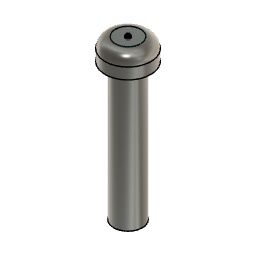
Trammel Toy Assembly (Autodesk Fusion 360 archive; units mm, degrees)
design "Screw"
Autodesk Fusion 360 part; units mm, degrees
sketch "Sketch1" plane through (0, 0, 0) normal (0, 0, 1) x (1, 0, 0)
  circle A0 centre (6.3408, 6.3573) radius 2.1209
  dimension "d1" = 4.2418
  measures "d1" diameter of A0
extrude "Extrude1" add sketch "Sketch1" along normal blind 20.32
sketch "Sketch6" plane through (0, 0, 20.32) normal (0, 0, 1) x (-1, 0, 0)
  circle A0 centre (-6.3408, -6.3573) radius 2.1209
  circle A1 centre (-6.3408, -6.3573) radius 3.3909
  point P0 (-6.3408, -6.3573)
  dimension "d7" = 6.7818
  constraint concentric A0 A1
  measures "d7" diameter of A1
extrude "Extrude2" add sketch "Sketch6" along normal blind 3.175 contours A0 | A1
fillet "Fillet1" radius 1.524 1 edges at (9.5022, 7.5835, 23.495)
sketch "Sketch7" plane through (0, 0, 23.495) normal (0, 0, 1) x (-1, 0, 0)
  circle A0 centre (-6.3408, -6.3573) radius 1.8669
  point P0 (-6.3408, -6.3573)
  constraint coincident P0 A0.centre

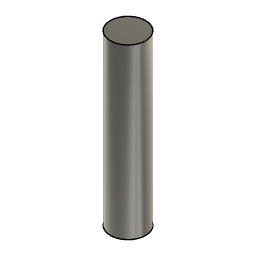
design "PIN"
Autodesk Fusion 360 part; units mm, degrees
sketch "Sketch1" plane through (0, 0, 0) normal (0, 0, 1) x (1, 0, 0)
  circle A0 centre (6.3408, 6.3573) radius 2.1209
  dimension "d1" = 4.2418
  measures "d1" diameter of A0
extrude "Extrude1" add sketch "Sketch1" along normal blind 20.32

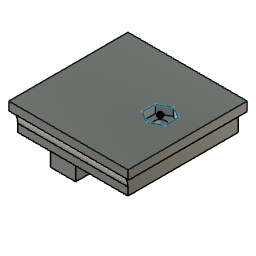
design "Trammel T1 v0"
Autodesk Fusion 360 part; units mm, degrees
sketch "Sketch1" plane through (0, 0, 0) normal (0, 0, 1) x (1, 0, 0)
  line L0 (0, 0) -> (53.975, 0)
  line L1 (53.975, 0) -> (53.975, 53.975)
  line L2 (53.975, 53.975) -> (0, 53.975)
  line L3 (0, 53.975) -> (0, 0)
  dimension "d1" = 53.975
  dimension "d2" = 53.975
  constraint horizontal L0
  constraint vertical L1
  constraint horizontal L2
  constraint vertical L3
  constraint coincident L0.start L3.end
  measures "d1" distance of L0.start L2.end
  measures "d2" distance of L0.start L0.end
extrude "Extrude1" add sketch "Sketch1" along normal blind 12.7
sketch "Sketch2" plane through (53.975, 0, 0) normal (1, 0, 0) x (0, 1, 0)
  line L0 (0, 0) -> (53.975, 0)
  line L1 (53.975, 0) -> (53.975, 12.7)
  line L2 (53.975, 12.7) -> (0, 12.7)
  line L3 (0, 12.7) -> (0, 0)
  line L4 (5.9309, 12.7) -> (0, 12.7)
  line L5 (0, 0) -> (0, 12.7)
  line L6 (0, 0) -> (9.5123, 0)
  line L7 (9.5123, 0) -> (9.5123, 3.175)
  line L8 (5.9309, 9.2761) -> (5.9309, 12.7)
  arc A0 (9.5123, 3.175) -> (5.9309, 9.2761) centre (2.5249, 3.175) ccw
  point P0 (5.9309, 12.7)
  point P1 (9.5123, 0)
  point P2 (9.5123, 3.175)
  point P3 (5.9309, 9.2761)
  dimension "d5" = 5.9309
  dimension "d6" = 9.5123
  dimension "d7" = 3.175
  dimension "d8" = 3.4239
  constraint coincident L2 P0
  constraint coincident L0.start L3.end
  constraint coincident L0 P1
  constraint coincident P0 L4.start
  constraint coincident L2.end L3.start
  constraint coincident P1 L6.end
  constraint coincident P2 L7.end
  constraint perpendicular L6 L7
  constraint coincident P3 L8.start
  constraint perpendicular L2 L8
  constraint tangent L7 A0
  measures "d5" distance of L2.end P0
  measures "d6" distance of L0.start P1
  measures "d7" distance of P1 P2
  measures "d8" distance of P0 P3
extrude "Extrude2" cut sketch "Sketch2" against normal blind 53.975 contours L0 L2 L3 L4 L5 L6 L7 L8 A0
sketch "Sketch3" plane through (0, 53.975, 0) normal (0, 1, 0) x (-1, 0, 0)
  line L0 (-53.975, 0) -> (0, 0)
  line L1 (0, 0) -> (0, 12.7)
  line L2 (0, 12.7) -> (-53.975, 12.7)
  line L3 (-53.975, 12.7) -> (-53.975, 0)
  line L4 (-48.0441, 12.7) -> (-53.975, 12.7)
  line L5 (-53.975, 0) -> (-44.4627, 0)
  line L6 (-44.4627, 9.017) -> (-44.4627, 0)
  line L7 (-44.4627, 9.017) -> (-48.0441, 9.017)
  line L8 (-48.0441, 9.017) -> (-48.0441, 12.7)
  point P0 (-48.0441, 12.7)
  point P1 (-44.4627, 0)
  point P2 (-44.4627, 9.017)
  point P3 (-48.0441, 12.7)
  point P4 (-44.4627, 9.017)
  point P5 (-48.0441, 9.017)
  dimension "d11" = 5.9309
  dimension "d12" = 9.5123
  dimension "d13" = 9.017
  constraint coincident L2 P3
  constraint coincident L0 P1
  constraint coincident P3 P0
  constraint coincident P4 P2
  constraint coincident L2.end L3.start
  constraint coincident L0.start L3.end
  constraint coincident P1 L5.end
  constraint perpendicular L5 L6
  constraint coincident P5 L7.end
  constraint perpendicular L6 L7
  constraint perpendicular L4 L8
  measures "d11" distance of L2.end P3
  measures "d12" distance of L0.start L5.end
  measures "d13" distance of P1 P4
extrude "Extrude3" cut sketch "Sketch3" against normal blind 53.975 contours L0 L2 L3 L4 L5 L6 L7 L8
sketch "Sketch4" plane through (0, 0, 0) normal (0, 0, -1) x (1, 0, 0)
  line L0 (44.4627, -53.975) -> (44.4627, -9.5123)
  line L1 (44.4627, -9.5123) -> (0, -9.5123)
  line L2 (0, -9.5123) -> (0, -53.975)
  line L3 (0, -53.975) -> (44.4627, -53.975)
  line L4 (12.7, -53.975) -> (22.86, -53.975)
  line L5 (22.86, -53.975) -> (22.86, -10.033)
  line L6 (22.86, -10.033) -> (12.7, -10.033)
  line L7 (12.7, -10.033) -> (12.7, -53.975)
  dimension "d16" = 43.942
  dimension "d17" = 10.16
  dimension "d18" = 12.7
  constraint horizontal L4
  constraint vertical L5
  constraint horizontal L6
  constraint vertical L7
  constraint coincident L3 L4.start
  measures "d16" distance of L4.start L6.end
  measures "d17" distance of L4.start L4.end
  measures "d18" distance of L2.end L4.start
sketch "Sketch5" plane through (0, 0, 12.7) normal (0, 0, 1) x (-1, 0, 0)
  line L0 (-48.0441, -5.9309) -> (-48.0441, -53.975)
  line L1 (-48.0441, -53.975) -> (0, -53.975)
  line L2 (0, -53.975) -> (0, -5.9309)
  line L3 (0, -5.9309) -> (-48.0441, -5.9309)
  line L4 (-39.9669, -34.292) -> (-35.3441, -36.9609)
  line L5 (-35.3441, -36.9609) -> (-30.7213, -34.292)
  line L6 (-30.7213, -34.292) -> (-30.7213, -28.954)
  line L7 (-30.7213, -28.954) -> (-35.3441, -26.2851)
  line L8 (-35.3441, -26.2851) -> (-39.9669, -28.954)
  line L9 (-39.9669, -28.954) -> (-39.9669, -34.292)
  point P0 (-35.3441, -31.623)
  point P1 (-35.3441, -31.623)
  dimension "d30" = 12.7
  dimension "d31" = 22.352
  dimension "d35" = 9.2456
  constraint coincident P1 P0
  measures "d30" distance of L0 P1
  measures "d31" distance of L1 P1
  measures "d35" distance of L6 L9
extrude "Extrude6" cut sketch "Sketch5" against normal blind 3.175 contours L4 L5 L6 L7 L8 L9
hole "Hole3" at (35.3441, 31.623, 12.7) direction (0, 0, -1) diameter 4.4958 depth 12.7 tip angle 118
extrude "Extrude7" add sketch "Sketch4" along normal blind 6.096 contours L3 L4 L5 L6 L7
equation "d27 = ( 0.364 / 2 ) * 1 in"

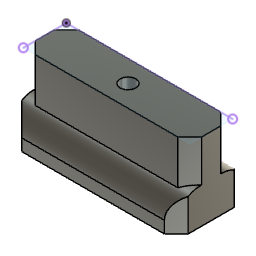
design "Pin Slider"
Autodesk Fusion 360 part; units mm, degrees
sketch "Sketch1" plane through (0, 0, 0) normal (0, 0, 1) x (1, 0, 0)
  line L0 (0, 0) -> (44.45, 0)
  line L1 (44.45, 0) -> (44.45, 18.6436)
  line L2 (44.45, 18.6436) -> (0, 18.6436)
  line L3 (0, 18.6436) -> (0, 0)
  dimension "d1" = 18.6436
  dimension "d2" = 44.45
  constraint horizontal L0
  constraint vertical L1
  constraint horizontal L2
  constraint vertical L3
  constraint coincident L0.start L3.end
  measures "d1" distance of L0.start L2.end
  measures "d2" distance of L1.end L2.end
extrude "Extrude1" add sketch "Sketch1" along normal blind 20.6502
sketch "Sketch2" plane through (0, 0, 20.6502) normal (0, 0, 1) x (-1, 0, 0)
  line L0 (0, -18.6436) -> (0, 0)
  line L1 (0, 0) -> (-44.45, 0)
  line L2 (-44.45, 0) -> (-44.45, -18.6436)
  line L3 (-44.45, -18.6436) -> (0, -18.6436)
  line L4 (0, -15.0622) -> (-44.45, -15.0622)
  line L5 (-44.45, -15.0622) -> (-44.45, -18.6436)
  line L6 (-44.45, -18.6436) -> (0, -18.6436)
  line L7 (0, -18.6436) -> (0, -15.0622)
  line L8 (0, -3.5814) -> (-44.45, -3.5814)
  line L9 (-44.45, -3.5814) -> (-44.45, 0)
  line L10 (-44.45, 0) -> (0, 0)
  line L11 (0, 0) -> (0, -3.5814)
  point P0 (0, -3.5814)
  point P1 (0, -18.6436)
  point P2 (0, -15.0622)
  dimension "d5" = 3.5814
  dimension "d6" = 3.5814
  constraint coincident L0 P0
  constraint coincident L0.start L3.end
  constraint coincident L0 P2
  constraint horizontal L4
  constraint vertical L5
  constraint horizontal L6
  constraint vertical L7
  constraint coincident L2.end L3.start
  constraint coincident P2 L4.start
  constraint horizontal L8
  constraint vertical L9
  constraint horizontal L10
  constraint vertical L11
  constraint coincident L1.end L2.start
  constraint coincident P0 L8.start
  measures "d5" distance of L0.end P0
  measures "d6" distance of P1 P2
extrude "Extrude2" cut sketch "Sketch2" against normal blind 11.1252 contours L0 L2 L3 L4 L5 L6 L7 | L0 L1 L2 L8 L9 L10 L11
sketch "Sketch3" plane through (0, 0, 20.6502) normal (0, 0, 1) x (-1, 0, 0)
  line L0 (0, -3.5814) -> (-44.45, -3.5814)
  line L1 (-44.45, -3.5814) -> (-44.45, -15.0622)
  line L2 (-44.45, -15.0622) -> (0, -15.0622)
  line L3 (0, -15.0622) -> (0, -3.5814)
sketch "Sketch4" plane through (0, 0, 0) normal (0, 1, 0) x (1, 0, 0)
chamfer "Chamfer1" distance 3.175 angle 45 1 edges at (44.45, 3.5814, 15.0876)
chamfer "Chamfer2" distance 3.175 angle 45 1 edges at (44.45, 0, 4.7625)
chamfer "Chamfer3" distance 3.175 angle 45 1 edges at (44.45, 15.0622, 15.0876)
chamfer "Chamfer4" distance 3.175 angle 45 1 edges at (44.45, 18.6436, 4.7625)
chamfer "Chamfer5" distance 3.175 angle 45 1 edges at (0, 18.6436, 4.7625)
chamfer "Chamfer6" distance 3.175 angle 45 3 edges at (0, 15.0622, 15.0876) (0, 3.5814, 15.0876) (0, 0, 4.7625)
fillet "Fillet1" radius 6.35 1 edges at (22.225, 0, 9.525)
fillet "Fillet2" radius 6.35 1 edges at (22.225, 18.6436, 9.525)
sketch "Sketch5" plane through (0, 0, 20.6502) normal (0, 0, 1) x (-1, 0, 0)
  line L0 (0, -15.0622) -> (0, -3.5814)
  line L1 (-44.45, -15.0622) -> (0, -15.0622)
sketch "Sketch6" plane through (0, 0, 0) normal (0, 0, -1) x (1, 0, 0)
  line L0 (3.175, 0) -> (0, -3.175)
  line L1 (0, -3.175) -> (0, -15.4686)
  line L2 (0, -15.4686) -> (3.175, -18.6436)
  line L3 (3.175, -18.6436) -> (41.275, -18.6436)
  line L4 (41.275, -18.6436) -> (44.45, -15.4686)
  line L5 (44.45, -15.4686) -> (44.45, -3.175)
  line L6 (44.45, -3.175) -> (41.275, 0)
  line L7 (41.275, 0) -> (3.175, 0)
  point P0 (22.225, -9.3218)
  dimension "d21" = 22.225
  dimension "d22" = 9.3218
  measures "d21" distance of L1 P0
  measures "d22" distance of L7 P0
hole "Hole1" at (22.225, 9.3218, 0) direction (0, 0, 1) diameter 4.191 depth 20.6502 tip angle 118 counterbore diameter 4.4958 counterbore depth 16.0782
equation "d7 = -0.813 in + 0.375 in"

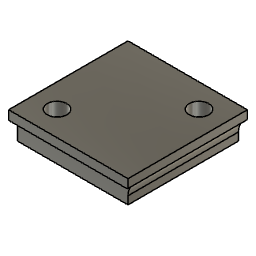
design "T24"
Autodesk Fusion 360 part; units mm, degrees
sketch "Sketch1" plane through (0, 0, 0) normal (0, 0, 1) x (1, 0, 0)
  line L0 (0, 0) -> (53.975, 0)
  line L1 (53.975, 0) -> (53.975, 53.975)
  line L2 (53.975, 53.975) -> (0, 53.975)
  line L3 (0, 53.975) -> (0, 0)
  dimension "d1" = 53.975
  dimension "d2" = 53.975
  constraint horizontal L0
  constraint vertical L1
  constraint horizontal L2
  constraint vertical L3
  constraint coincident L0.start L3.end
  measures "d1" distance of L0.start L0.end
  measures "d2" distance of L0.start L2.end
extrude "Extrude1" add sketch "Sketch1" along normal blind 12.7
sketch "Sketch2" plane through (0, 0, 0) normal (0, -1, 0) x (1, 0, 0)
  line L0 (0, 0) -> (53.975, 0)
  line L1 (53.975, 0) -> (53.975, 12.7)
  line L2 (53.975, 12.7) -> (0, 12.7)
  line L3 (0, 12.7) -> (0, 0)
  line L4 (44.4627, 0) -> (44.4627, 3.175)
  line L5 (44.4627, 3.175) -> (44.4627, 0)
  line L6 (53.975, 0) -> (44.4627, 0)
  line L7 (53.975, 0) -> (53.975, 12.7)
  line L8 (48.0441, 12.7) -> (53.975, 12.7)
  line L9 (48.0441, 12.7) -> (48.0441, 9.2761)
  arc A0 (48.0441, 9.2761) -> (44.4627, 3.175) centre (51.4501, 3.175) ccw
  point P0 (44.4627, 0)
  point P1 (48.0441, 12.7)
  point P2 (53.975, 12.7)
  point P3 (48.0441, 9.2761)
  point P4 (44.4627, 3.175)
  dimension "d5" = 9.5123
  dimension "d6" = 5.9309
  dimension "d7" = 3.175
  dimension "d8" = 3.4239
  dimension "d9" = 6.9874
  constraint coincident L0 P0
  constraint coincident L2 P1
  constraint coincident P2 L1.end
  constraint coincident P0 L4.start
  constraint coincident P4 L4.end
  constraint perpendicular L0 L4
  constraint coincident L0.end L1.start
  constraint coincident P1 L8.start
  constraint coincident P3 L9.end
  constraint perpendicular L8 L9
  constraint tangent L4 A0
  measures "d5" distance of L0.end P0
  measures "d6" distance of P1 P2
  measures "d7" distance of P0 P4
  measures "d8" distance of P1 P3
  measures "d9" radius of A0
extrude "Extrude2" cut sketch "Sketch2" against normal blind 53.975 contours L0 L1 L2 L4 L5 L6 L7 L8 L9 A0
sketch "Sketch3" plane through (0, 0, 0) normal (1, 0, 0) x (0, 1, 0)
  line L0 (9.5123, 0) -> (9.5123, 9.017)
  line L1 (9.5123, 9.017) -> (5.9309, 9.017)
  line L2 (5.9309, 9.017) -> (5.9309, 12.7)
  line L3 (5.9309, 12.7) -> (0, 12.7)
  line L4 (0, 12.7) -> (0, 0)
  line L5 (0, 0) -> (9.5123, 0)
  point P0 (9.5123, 0)
  point P1 (9.5123, 0)
  point P2 (9.5123, 9.017)
  point P3 (9.5123, 9.017)
  point P4 (0, 12.7)
  point P5 (0, 12.7)
  point P6 (5.9309, 12.7)
  point P7 (9.5123, 9.017)
  point P8 (5.9309, 12.7)
  point P9 (5.9309, 9.017)
  dimension "d12" = 9.5123
  dimension "d13" = 9.017
  dimension "d15" = 5.9309
  constraint coincident L4.end L5.start
  constraint coincident P1 P0
  constraint coincident P3 P2
  constraint coincident P5 P4
  constraint coincident P8 P6
  constraint coincident P7 P3
  constraint vertical L0
  constraint coincident P9 L1.end
  constraint perpendicular L0 L1
  constraint perpendicular L1 L2
  constraint perpendicular L0 L3
  constraint perpendicular L0 L5
  measures "d12" distance of L4.end P1
  measures "d13" distance of P1 P7
  measures "d15" distance of P5 P8
extrude "Extrude3" cut sketch "Sketch3" along normal blind 53.975
sketch "Sketch4" plane through (0, 0, 12.7) normal (0, 0, 1) x (-1, 0, 0)
  line L0 (0, -5.9309) -> (-48.0441, -5.9309)
  line L1 (-48.0441, -5.9309) -> (-48.0441, -53.975)
  line L2 (-48.0441, -53.975) -> (0, -53.975)
  line L3 (0, -53.975) -> (0, -5.9309)
  point P0 (-9.525, -15.875)
  point P1 (-38.1, -44.45)
  dimension "d18" = 9.525
  dimension "d19" = 38.1
  dimension "d20" = 9.525
  dimension "d21" = 38.1
  measures "d18" distance of L3 P0
  measures "d19" vertical distance of L2.end P0
  measures "d20" distance of L2 P1
  measures "d21" distance of L3 P1
hole "Hole1" at (9.525, 15.875, 12.7) at (38.1, 44.45, 12.7) direction (0, 0, -1) diameter 4.4958 depth 12.7 tip angle 118 counterbore diameter 7.874 counterbore depth 5.3848

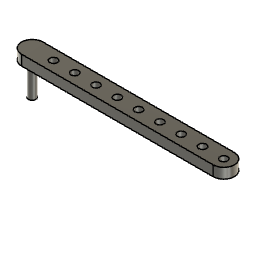
design "Handle"
Autodesk Fusion 360 part; units mm, degrees
sketch "Sketch1" plane through (0, 0, 0) normal (0, 0, 1) x (1, 0, 0)
  line L0 (0, 0) -> (127, 0)
  line L1 (127, 0) -> (127, 12.7)
  line L2 (127, 12.7) -> (0, 12.7)
  line L3 (0, 12.7) -> (0, 0)
  dimension "d1" = 127
  dimension "d2" = 12.7
  constraint horizontal L0
  constraint vertical L1
  constraint horizontal L2
  constraint vertical L3
  constraint coincident L0.start L3.end
  measures "d1" distance of L0.start L0.end
  measures "d2" distance of L0.start L2.end
extrude "Extrude1" add sketch "Sketch1" along normal blind 6.096
fillet "Fillet1" radius 6.35 4 edges at (127, 0, 3.048) (127, 12.7, 3.048) (0, 12.7, 3.048) (0, 0, 3.048)
sketch "Sketch2" plane through (0, 0, 6.096) normal (0, 0, 1) x (-1, 0, 0)
  arc A0 (-6.35, -12.7) -> (-6.35, 0) centre (-6.35, -6.35) ccw
  line L0 (-6.35, 0) -> (-120.65, 0)
  arc A1 (-120.65, 0) -> (-120.65, -12.7) centre (-120.65, -6.35) ccw
  line L1 (-120.65, -12.7) -> (-6.35, -12.7)
  circle A2 centre (-6.35, -6.35) radius 2.2479
  point P0 (-6.35, -6.35)
  point P1 (-6.35, -6.35)
  point P2 (-19.05, -6.35)
  point P3 (-19.05, -6.35)
  point P4 (-31.75, -6.35)
  point P5 (-31.75, -6.35)
  point P6 (-44.45, -6.35)
  point P7 (-44.45, -6.35)
  point P8 (-57.15, -6.35)
  point P9 (-57.15, -6.35)
  point P10 (-69.85, -6.35)
  point P11 (-69.85, -6.35)
  point P12 (-82.55, -6.35)
  point P13 (-95.25, -6.35)
  point P14 (-107.95, -6.35)
  point P15 (-120.65, -6.35)
  dimension "d7" = 12.7
  dimension "d8" = 12.7
  dimension "d9" = 12.7
  dimension "d10" = 12.7
  dimension "d11" = 12.7
  dimension "d12" = 12.7
  dimension "d13" = 12.7
  dimension "d14" = 12.7
  dimension "d15" = 12.7
  dimension "d20" = 4.4958
  constraint coincident P1 P0
  constraint coincident P3 P2
  constraint coincident P5 P4
  constraint coincident P7 P6
  constraint coincident P9 P8
  constraint coincident P11 P10
  constraint coincident P15 A1.centre
  measures "d7" distance of P1 P3
  measures "d8" distance of P3 P5
  measures "d9" distance of P5 P7
  measures "d10" distance of P7 P9
  measures "d11" distance of P9 P11
  measures "d12" distance of P11 P12
  measures "d13" distance of P12 P13
  measures "d14" distance of P13 P14
  measures "d15" distance of P14 P15
  measures "d20" diameter of A2
hole "Hole1" at (107.95, 6.35, 6.096) at (120.65, 6.35, 6.096) at (82.55, 6.35, 6.096) at (95.25, 6.35, 6.096) at (69.85, 6.35, 6.096) at (57.15, 6.35, 6.096) at (44.45, 6.35, 6.096) at (31.75, 6.35, 6.096) at (31.75, 6.35, 6.096) at (6.35, 6.35, 6.096) at (19.05, 6.35, 6.096) direction (0, 0, -1) diameter 4.4958 depth 6.096 tip angle 118
sketch "Sketch4" plane through (0, 0, 0) normal (0, 0, 1) x (1, 0, 0)
extrude "Extrude2" add sketch "Sketch2" against normal blind 25.4 contours A2

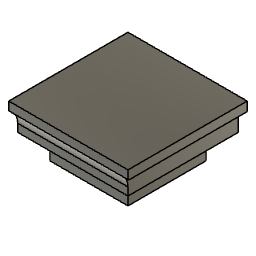
design "Trammel T3 C v0"
Autodesk Fusion 360 part; units mm, degrees
sketch "Sketch1" plane through (0, 0, 0) normal (0, 0, 1) x (1, 0, 0)
  line L0 (0, 0) -> (53.975, 0)
  line L1 (53.975, 0) -> (53.975, 53.975)
  line L2 (53.975, 53.975) -> (0, 53.975)
  line L3 (0, 53.975) -> (0, 0)
  dimension "d1" = 53.975
  dimension "d2" = 53.975
  constraint horizontal L0
  constraint vertical L1
  constraint horizontal L2
  constraint vertical L3
  constraint coincident L0.start L3.end
  measures "d1" distance of L0.start L2.end
  measures "d2" distance of L1.end L2.end
extrude "Extrude1" add sketch "Sketch1" along normal blind 12.7
sketch "Sketch2" plane through (53.975, 0, 0) normal (1, 0, 0) x (0, 1, 0)
  line L0 (0, 0) -> (53.975, 0)
  line L1 (53.975, 0) -> (53.975, 12.7)
  line L2 (53.975, 12.7) -> (0, 12.7)
  line L3 (0, 12.7) -> (0, 0)
  line L4 (9.5123, 0) -> (9.5123, 3.175)
  line L5 (5.9309, 12.7) -> (0, 12.7)
  line L6 (5.9309, 9.2761) -> (5.9309, 12.7)
  line L7 (0, 0) -> (0, 12.7)
  line L8 (0, 0) -> (9.5123, 0)
  arc A0 (9.5123, 3.175) -> (5.9309, 9.2761) centre (2.5249, 3.175) ccw
  point P0 (5.9309, 12.7)
  point P1 (9.5123, 0)
  point P2 (9.5123, 3.175)
  point P3 (5.9309, 9.2761)
  dimension "d5" = 5.9309
  dimension "d6" = 9.5123
  dimension "d7" = 3.175
  dimension "d8" = 3.4239
  dimension "d9" = 6.9874
  constraint coincident L2 P0
  constraint coincident L0 P1
  constraint coincident P1 L4.start
  constraint coincident P2 L4.end
  constraint perpendicular L0 L4
  constraint coincident P0 L5.start
  constraint coincident L2.end L3.start
  constraint coincident P3 L6.start
  constraint perpendicular L5 L6
  constraint coincident L0.start L3.end
  constraint tangent L4 A0
  measures "d5" distance of L2.end P0
  measures "d6" distance of L0.start L4.start
  measures "d7" distance of P1 P2
  measures "d8" distance of P0 P3
  measures "d9" radius of A0
extrude "Extrude2" cut sketch "Sketch2" against normal blind 53.975 contours L0 L2 L3 L4 L5 L6 L7 L8 A0
sketch "Sketch3" plane through (0, 53.975, 0) normal (0, 1, 0) x (-1, 0, 0)
  line L0 (-53.975, 0) -> (0, 0)
  line L1 (0, 0) -> (0, 12.7)
  line L2 (0, 12.7) -> (-53.975, 12.7)
  line L3 (-53.975, 12.7) -> (-53.975, 0)
  line L4 (-44.4627, 0) -> (-44.4627, 9.017)
  line L5 (-48.0441, 9.017) -> (-48.0441, 12.7)
  line L6 (-48.0441, 9.017) -> (-44.4627, 9.017)
  line L7 (-48.0441, 12.7) -> (-53.975, 12.7)
  line L8 (-53.975, 0) -> (-53.975, 12.7)
  line L9 (-44.4627, 0) -> (-53.975, 0)
  point P0 (-48.0441, 12.7)
  point P1 (-44.4627, 0)
  point P2 (-44.4627, 0)
  point P3 (-44.4627, 9.017)
  point P4 (-48.0441, 9.017)
  dimension "d12" = 5.9309
  dimension "d13" = 9.5123
  dimension "d14" = 9.017
  constraint coincident L2 P0
  constraint coincident L0 P2
  constraint coincident P2 P1
  constraint coincident P3 L4.end
  constraint perpendicular L0 L4
  constraint coincident P4 L5.start
  constraint coincident P0 L5.end
  constraint perpendicular L2 L5
  constraint perpendicular L4 L6
  constraint coincident L2.end L3.start
  constraint coincident L0.start L3.end
  measures "d12" distance of L2.end P0
  measures "d13" distance of L0.start P2
  measures "d14" distance of P2 P3
extrude "Extrude3" cut sketch "Sketch3" against normal blind 53.975 contours L0 L2 L3 L4 L5 L6 L7 L8 L9
sketch "Sketch4" plane through (0, 0, 0) normal (0, 0, -1) x (1, 0, 0)
  line L0 (44.4627, -53.975) -> (44.4627, -9.5123)
  line L1 (44.4627, -9.5123) -> (0, -9.5123)
  line L2 (0, -9.5123) -> (0, -53.975)
  line L3 (0, -53.975) -> (44.4627, -53.975)
  line L4 (10.3124, -43.6626) -> (41.8084, -43.6626)
  line L5 (41.8084, -43.6626) -> (41.8084, -12.1666)
  line L6 (41.8084, -12.1666) -> (10.3124, -12.1666)
  line L7 (10.3124, -12.1666) -> (10.3124, -43.6626)
  dimension "d17" = 31.496
  dimension "d18" = 31.496
  dimension "d19" = 10.3124
  dimension "d20" = 10.3124
  constraint horizontal L4
  constraint vertical L5
  constraint horizontal L6
  constraint vertical L7
  measures "d17" distance of L4.start L6.end
  measures "d18" distance of L4.start L4.end
  measures "d19" distance of L2 L4.start
  measures "d20" distance of L3 L4.start
extrude "Extrude4" add sketch "Sketch4" along normal blind 6.096 contours L4 L5 L6 L7

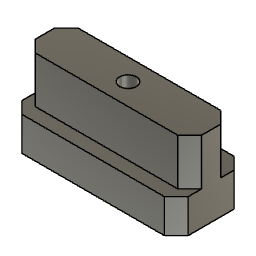
design "Screw Slider Block"
Autodesk Fusion 360 part; units mm, degrees
sketch "Sketch1" plane through (0, 0, 0) normal (0, 0, 1) x (1, 0, 0)
  line L0 (0, 0) -> (-44.45, 0)
  line L1 (-44.45, 0) -> (-44.45, 18.6436)
  line L2 (-44.45, 18.6436) -> (0, 18.6436)
  line L3 (0, 18.6436) -> (0, 0)
  dimension "d1" = 44.45
  dimension "d2" = 18.6436
  constraint horizontal L0
  constraint vertical L1
  constraint horizontal L2
  constraint vertical L3
  constraint coincident L0.start L3.end
  measures "d1" distance of L1.end L2.end
  measures "d2" distance of L0.end L1.end
extrude "Extrude1" add sketch "Sketch1" along normal blind 21.4376
sketch "Sketch2" plane through (0, 0, 21.4376) normal (0, 0, 1) x (-1, 0, 0)
  line L0 (0, -18.6436) -> (44.45, -18.6436)
  line L1 (44.45, -18.6436) -> (44.45, 0)
  line L2 (44.45, 0) -> (0, 0)
  line L3 (0, 0) -> (0, -18.6436)
  line L4 (0, -18.6436) -> (44.45, -18.6436)
  line L5 (44.45, -18.6436) -> (44.45, -15.0622)
  line L6 (44.45, -15.0622) -> (0, -15.0622)
  line L7 (0, -15.0622) -> (0, -18.6436)
  line L8 (0, 0) -> (44.45, 0)
  line L9 (44.45, 0) -> (44.45, -3.5814)
  line L10 (44.45, -3.5814) -> (0, -3.5814)
  line L11 (0, -3.5814) -> (0, 0)
  dimension "d5" = 3.5814
  dimension "d6" = 3.5814
  constraint horizontal L4
  constraint vertical L5
  constraint horizontal L6
  constraint vertical L7
  constraint coincident L1 L5.end
  constraint coincident L0.start L3.end
  constraint horizontal L8
  constraint vertical L9
  constraint horizontal L10
  constraint vertical L11
  constraint coincident L1 L9.end
  constraint coincident L2.end L3.start
  measures "d5" distance of L0.start L6.end
  measures "d6" distance of L2.end L10.end
extrude "Extrude2" cut sketch "Sketch2" against normal blind 12.4206 contours L1 L2 L3 L8 L9 L10 L11
extrude "Extrude3" cut sketch "Sketch2" against normal blind 12.4206 contours L0 L1 L3 L4 L5 L6 L7
chamfer "Chamfer1" distance 3.175 angle 45 8 edges at (0, 3.5814, 15.2273) (0, 15.0622, 15.2273) (0, 0, 4.5085) (0, 18.6436, 4.5085) (-44.45, 0, 4.5085) (-44.45, 3.5814, 15.2273) (-44.45, 15.0622, 15.2273) (-44.45, 18.6436, 4.5085)
sketch "Sketch3" plane through (0, 0, 21.4376) normal (0, 0, 1) x (-1, 0, 0)
  line L0 (41.275, -15.0622) -> (44.45, -11.8872)
  line L1 (44.45, -11.8872) -> (44.45, -6.7564)
  line L2 (44.45, -6.7564) -> (41.275, -3.5814)
  line L3 (41.275, -3.5814) -> (3.175, -3.5814)
  line L4 (3.175, -3.5814) -> (0, -6.7564)
  line L5 (0, -6.7564) -> (0, -11.8872)
  line L6 (0, -11.8872) -> (3.175, -15.0622)
  line L7 (3.175, -15.0622) -> (41.275, -15.0622)
  line L8 (3.175, 0) -> (41.275, 0)
  point P0 (22.225, -9.3218)
  point P1 (22.225, -9.3218)
  dimension "d12" = 9.3218
  dimension "d13" = 22.225
  constraint coincident P1 P0
  measures "d12" distance of P1 L8
  measures "d13" distance of L5 P1
hole "Hole1" at (-22.225, 9.3218, 21.4376) direction (0, 0, -1) diameter 4.4958 depth 21.4376 tip angle 118
sketch "Sketch5" plane through (0, 0, 0) normal (0, 0, -1) x (1, 0, 0)
  circle A0 centre (-22.225, -9.3218) radius 2.2479
  line L0 (-44.45, -15.4686) -> (-41.275, -18.6436)
  line L1 (-41.275, -18.6436) -> (-3.175, -18.6436)
  line L2 (-3.175, -18.6436) -> (0, -15.4686)
  line L3 (0, -15.4686) -> (0, -3.175)
  line L4 (0, -3.175) -> (-3.175, 0)
  line L5 (-3.175, 0) -> (-41.275, 0)
  line L6 (-41.275, 0) -> (-44.45, -3.175)
  line L7 (-44.45, -3.175) -> (-44.45, -15.4686)
  line L8 (-25.0553, -4.4196) -> (-27.8856, -9.3218)
  line L9 (-27.8856, -9.3218) -> (-25.0553, -14.224)
  line L10 (-25.0553, -14.224) -> (-19.3947, -14.224)
  line L11 (-19.3947, -14.224) -> (-16.5644, -9.3218)
  line L12 (-16.5644, -9.3218) -> (-19.3947, -4.4196)
  line L13 (-19.3947, -4.4196) -> (-25.0553, -4.4196)
  point P0 (-22.225, -9.3218)
  point P1 (-22.225, -9.3218)
  dimension "d18" = 4.9022
  constraint coincident P0 A0.centre
  constraint coincident P1 P0
  measures "d18" distance of P1 L13
extrude "Extrude4" cut sketch "Sketch5" against normal blind 6.477 contours L8 L9 L10 L11 L12 L13
equation "d7 = 0.355 in - 0.844 in"
equation "d9 = 0.355 in - 0.844 in"
equation "d18 = ( 0.386 / 2 ) * 1 in"
